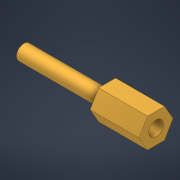
# Autodesk Inventor part: ArchSpacer
Saved by Autodesk Inventor 2022 (Build 260153000, 153)
## iProperties
Created: 2022-04-02
Part Number: ArchSpacer
Material: Brass, Soft Yellow
Document SubType Name: Modeling
Designer: Sergei
Density: 8.47 g/cm^3
Appearance: Brass - Satin
Author: Sergei
Autodesk Inventor part; units mm, degrees
ref_plane "YZ Plane" through (0, 0, 0) normal (1, 0, 0) x (0, 1, 0)
ref_plane "XZ Plane" through (0, 0, 0) normal (0, 1, 0) x (-1, 0, 0)
ref_plane "XY Plane" through (0, 0, 0) normal (0, 0, 1) x (1, 0, 0)
sketch "Sketch1" plane through (0, 0, 0) normal (1, 0, 0) x (0, 1, 0)
  line L0 (0.0055, 3.4536) -> (3.0055, 1.7216)
  line L1 (3.0055, 1.7216) -> (3.0055, -1.7425)
  line L2 (3.0055, -1.7425) -> (0.0055, -3.4746)
  line L3 (0.0055, -3.4746) -> (-2.9945, -1.7425)
  line L4 (-2.9945, -1.7425) -> (-2.9945, 1.7216)
  line L5 (-2.9945, 1.7216) -> (0.0055, 3.4536)
  point P0 (0.0055, -0.0105)
  dimension "d1" = 6
  constraints: 12 end point, 1 horizontal alignment, 1 vertical alignment, 13 other
  measures "d1" distance between parallel lines of L4 L1
extrude "Extrusion1" add sketch "Sketch1" along normal blind 10
sketch "Sketch2" plane through (0, 0, 0) normal (-1, 0, 0) x (0, 0, 1)
  circle A0 centre (0, 0) radius 1.5
  dimension "d4" = 3
  constraints: 1 centre point, 1 coincident
  measures "d4" diameter of A0
extrude "Extrusion2" add sketch "Sketch2" along normal blind 17
sketch "Sketch3" plane through (10, 0, 0) normal (1, 0, 0) x (0, 0, -1)
  circle A0 centre (0, 0) radius 1.5
  dimension "d7" = 3
  constraints: 1 centre point, 1 coincident
  measures "d7" diameter of A0
extrude "Extrusion3" cut sketch "Sketch3" against normal blind 6
body "Solid1"
